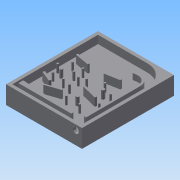
# Autodesk Inventor part: ball
Saved by Autodesk Inventor 2017 (Build 210142000, 142)
## iProperties
Created: 2018-01-03
Part Number: ball
Material: 一般
Document SubType Name: Modeling
Designer: user
Density: 1 g/cm^3
Appearance: 預設
Author: user
Autodesk Inventor part; units mm, degrees
ref_plane "YZ Plane" through (0, 0, 0) normal (1, 0, 0) x (0, 1, 0)
ref_plane "XZ Plane" through (0, 0, 0) normal (0, 1, 0) x (-1, 0, 0)
ref_plane "XY Plane" through (0, 0, 0) normal (0, 0, 1) x (1, 0, 0)
sketch "草圖1" plane through (0, 0, 0) normal (0, 1, 0) x (-1, 0, 0)
  line L0 (133, 0) -> (-133, 0) construction
  line L1 (0, -161) -> (0, 161) construction
  line L2 (95, -115) -> (-95, -115)
  line L3 (-95, -115) -> (-95, 115)
  line L4 (-95, 115) -> (95, 115)
  line L5 (95, 115) -> (95, -115)
  point P0 (0, 0)
  dimension "d0" = 190
  dimension "d1" = 230
  constraints: 8 end point, 2 parallel, 1 horizontal, 1 perpendicular, 2 other
  measures "d0" distance of L3.end L4.end
  measures "d1" distance of L2.end L3.end
extrude "擠出1" add sketch "草圖1" along normal blind 40
sketch "草圖3" plane through (0, 0, 0) normal (1, 0, 0) x (0, 1, 0)
  line L0 (0, 115) -> (0, -115) construction
  line L1 (0, 115) -> (40, 115) construction
  line L2 (40, -115) -> (40, 115) construction
  line L3 (0, -115) -> (40, -115) construction
  line L4 (-8, 0) -> (48, 0) construction
  line L5 (0, -161) -> (0, 161) construction
  line L6 (10, 107) -> (40, 107)
  line L7 (40, 107) -> (40, -107)
  line L8 (40, -107) -> (10, -107)
  line L9 (10, 107) -> (10, -107.0049)
  point P0 (0, 0)
  dimension "d13" = 8
  dimension "d14" = 8
  dimension "d27" = 10
  constraints: 8 end point, 3 perpendicular, 3 point on line, 1 parallel
  measures "d13" distance of L2.start L7.end
  measures "d14" vertical distance of L0.start L6.start
  measures "d27" distance between parallel lines of L0 L9
sketch "草圖2" plane through (0, 40, 0) normal (0, 1, 0) x (1, 0, 0)
  line L0 (95, 115) -> (-95, 115) construction
  line L1 (-95, 115) -> (-95, -115) construction
  line L2 (-95, -115) -> (95, -115) construction
  line L3 (95, -115) -> (95, 115) construction
  line L4 (-133, 0) -> (133, 0) construction
  line L5 (0, 161) -> (0, -161) construction
  line L6 (-87, 107) -> (87, 107)
  line L7 (87, 107) -> (87, -107)
  line L8 (87, -107) -> (-87, -107)
  line L9 (-87, -107) -> (-87, 107)
  line L10 (-87, -80.0748) -> (45.1402, -87)
  line L11 (45.1402, -92) -> (-87, -92)
  line L12 (45.1402, -92) -> (45.1402, -87)
  line L13 (72, 53.3199) -> (72, -81.708)
  line L14 (72, -81.708) -> (67, -81.708)
  line L15 (67, -81.708) -> (67, 53.3199)
  arc A0 (67, 53.3199) -> (43.2398, 73.9691) centre (46.1471, 53.3199) ccw
  arc A1 (72, 53.3199) -> (42.5427, 78.9203) centre (46.1471, 53.3199) ccw
  line L16 (43.2398, 73.9691) -> (33.9304, 72.6584)
  line L17 (45.4216, 79.3256) -> (33.2333, 77.6096)
  line L18 (33.2333, 77.6096) -> (33.9304, 72.6584)
  point P0 (0, 0)
  dimension "d4" = 8
  dimension "d5" = 15
  dimension "d6" = 5
  dimension "d7" = 3
  dimension "d8" = 15
  dimension "d9" = 5
  dimension "d10" = 5
  constraints: 26 end point, 5 perpendicular, 4 point on circle, 3 point on line, 3 tangent, 2 centre point, 2 parallel, 3 other
  measures "d4" distance between parallel lines of L0 L6
  measures "d5" distance between parallel lines of L8 L11
  measures "d6" distance of L10.end L11.start
  measures "d7" angle of L11 L10
  measures "d8" distance between parallel lines of L7 L13
  measures "d9" distance of L13.end L14.end
  measures "d10" radial gap between concentric circles of A0 A1
extrude "擠出7" cut sketch "草圖3" along normal mid plane 174
extrude "擠出8" add sketch "草圖2" against normal up to next contours L10 L12 L11 L9 | L13 L14 L15 A0 L16 L18 L17 A1
sketch "草圖6" plane through (-87, 10, 107) normal (0, 1, 0) x (1, 0, 0)
  line L0 (132.1402, 15) -> (0, 15) projected
  line L1 (0, 15) -> (0, 0) projected
  line L2 (0, 0) -> (174, 0) projected
  line L3 (174, 0) -> (174, 214) projected
  line L4 (0, 214) -> (174, 214) projected
  line L5 (0, 214) -> (0, 26.9252) projected
  line L6 (0, 26.9252) -> (132.1402, 20) projected
  line L7 (132.1402, 20) -> (132.1402, 15) projected
  arc A0 (159, 160.3199) -> (129.5427, 185.9203) centre (133.1471, 160.3199) ccw projected
  line L8 (159, 160.3199) -> (159, 25.292) projected
  line L9 (159, 25.292) -> (154, 25.292) projected
  line L10 (154, 25.292) -> (154, 160.3199) projected
  arc A1 (154, 160.3199) -> (130.2398, 180.9691) centre (133.1471, 160.3199) ccw projected
  line L11 (130.2398, 180.9691) -> (120.9304, 179.6584) projected
  line L12 (120.9304, 179.6584) -> (120.2333, 184.6096) projected
  line L13 (120.2333, 184.6096) -> (129.5427, 185.9203) projected
  point P0 (87, 107)
extrude "擠出9" add sketch "草圖6" along normal blind 15
sketch "草圖9" plane through (-95, 0, 115) normal (0, 0, 1) x (1, 0, 0)
  line L0 (182, 25) -> (8, 25) construction
  line L1 (182, 40) -> (182, 25) construction
  line L2 (167, 40) -> (167, 25) construction
  circle A0 centre (174.5, 32.5) radius 7.5
  point P0 (95, 0)
  dimension "d64" = 15
  constraints: 2 tangent, 1 centre point
  measures "d64" diameter of A0
extrude "擠出11" cut sketch "草圖9" against normal blind 20
sketch "草圖10" plane through (0, 40, 0) normal (0, 1, 0) x (1, 0, 0)
  line L0 (-87, -92) -> (45.1402, -92) construction
  line L1 (45.1402, -92) -> (45.1402, -87) construction
  line L2 (45.1402, -87) -> (-87, -80.0748) construction
  line L3 (-87, -80.0748) -> (-87, 107) projected
  line L4 (-87, 107) -> (87, 107) projected
  line L5 (87, 107) -> (87, -107) projected
  line L6 (87, -107) -> (79.5, -107) projected
  line L7 (79.5, -115) -> (79.5, -107) projected
  line L8 (79.5, -115) -> (95, -115) projected
  line L9 (95, -115) -> (95, 115) projected
  line L10 (95, 115) -> (-95, 115) projected
  line L11 (-95, 115) -> (-95, -115) projected
  line L12 (-95, -115) -> (79.5, -115) projected
  line L13 (79.5, -107) -> (-87, -107) projected
  line L14 (-87, -107) -> (-87, -92) projected
  line L15 (-87, -80.0748) -> (-87, -92)
  point P0 (0, 0)
  constraints: 2 end point, 1 vertical
extrude "擠出12" add sketch "草圖10" along normal blind 5
fillet "圓角1" radius 50 1 edges at (87, 35, -107)
sketch "草圖11" plane through (-87, 25, 107) normal (0, 1, 0) x (1, 0, 0)
  line L0 (16.0333, 148.1759) -> (51.7064, 141.7244)
  line L1 (51.7064, 141.7244) -> (50.8968, 137.2481)
  line L2 (50.8968, 137.2481) -> (15.2237, 143.6996)
  line L3 (15.2237, 143.6996) -> (16.0333, 148.1759)
  line L4 (182, 222) -> (-8, 222) projected
  line L5 (70.9047, 222) -> (70.9047, 192.887) construction
  line L6 (125.7761, 148.1759) -> (90.103, 141.7244)
  line L7 (90.103, 141.7244) -> (90.9126, 137.2481)
  line L8 (90.9126, 137.2481) -> (126.5857, 143.6996)
  line L9 (126.5857, 143.6996) -> (125.7761, 148.1759)
  circle A0 centre (26.1565, 124.5773) radius 2.5
  circle A1 centre (11.4824, 101.8214) radius 2.5
  circle A2 centre (23.8526, 77.7353) radius 2.5
  circle A3 centre (50.8968, 76.4051) radius 2.5
  circle A4 centre (65.5709, 99.161) radius 2.5
  circle A5 centre (53.2008, 123.2471) radius 2.5
  circle A6 centre (126.3016, 41.8829) radius 2.5
  circle A7 centre (149.3019, 68.1668) radius 2.5
  circle A8 centre (143.0928, 102.5369) radius 2.5
  circle A9 centre (112.3498, 119.1118) radius 2.5
  circle A10 centre (80.2231, 105.4102) radius 2.5
  circle A11 centre (70.9047, 71.7498) radius 2.5
  circle A12 centre (91.4116, 43.4775) radius 2.5
  line L10 (95.0789, 88.3359) -> (132.687, 78.9051)
  line L11 (132.687, 78.9051) -> (131.5197, 74.2498)
  line L12 (131.5197, 74.2498) -> (93.9116, 83.6806)
  line L13 (93.9116, 83.6806) -> (95.0789, 88.3359)
  line L14 (38.5267, 40.9775) -> (73.475, 52.9247)
  line L15 (73.475, 52.9247) -> (74.6702, 49.4284)
  line L16 (74.6702, 49.4284) -> (39.7219, 37.4812)
  line L17 (39.7219, 37.4812) -> (38.5267, 40.9775)
  line L18 (12.2608, 69.2526) -> (39.4354, 58.057)
  line L19 (39.4354, 58.057) -> (37.5308, 53.434)
  line L20 (37.5308, 53.434) -> (10.3562, 64.6295)
  line L21 (10.3562, 64.6295) -> (12.2608, 69.2526)
  circle A13 centre (106.3327, 56.6592) radius 4
  circle A14 centre (123.8016, 102.7619) radius 4
  circle A15 centre (27.1857, 95.1306) radius 3.3162
  circle A16 centre (48.3968, 105.4102) radius 2.6483
  point P0 (38.5267, 100.4912)
  point P1 (110.5122, 78.9051)
  dimension "d70" = 5
  dimension "d73" = 360
  dimension "d75" = 5
  dimension "d78" = 360
  dimension "d80" = 5
  dimension "d81" = 8
  dimension "d82" = 8
  constraints: 42 end point, 17 centre point, 10 perpendicular, 4 symmetric about line, 1 point on line, 1 vertical, 28 other
  measures "d70" diameter of A0
  measures "d75" diameter of A6
  measures "d80" distance between parallel lines of L18 L20
  measures "d81" diameter of A13
  measures "d82" diameter of A14
extrude "擠出13" add sketch "草圖11" along normal up to surface (20 mm away)
